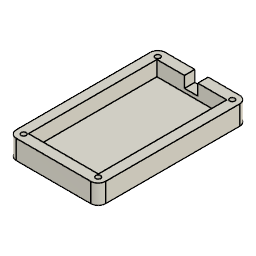
casemalumacropad (Autodesk Fusion 360 design; units mm, degrees)
part number: 2026-01-20-12-17-54-837
part number: 2026-01-20-12-22-16-145
part number: 2026-01-20-12-33-53-542
Autodesk Fusion 360 part; units mm, degrees
sketch "Esboço1" plane through (0, 0, 0) normal (0, 0, 1) x (1, 0, 0) in component "Case"
sketch "Esboço1 (2)" plane through (0, 0, 0) normal (0, 0, 1) x (1, 0, 0) in component "Component"
  line L0 (-33.5931, -33.1775) -> (13.2718, -33.1775)
  line L1 (13.2718, -33.1775) -> (13.2718, 52.9754)
  line L2 (13.2718, 52.9754) -> (-33.5931, 52.9754)
  line L3 (-33.5931, 52.9754) -> (-33.5931, -33.1775)
  line L4 (-40, 60) -> (20, 60)
  line L5 (20, 60) -> (20, -40)
  line L6 (20, -40) -> (-40, -40)
  line L7 (-40, -40) -> (-40, 60)
  circle A0 centre (-35, -35) radius 1.7
  circle A1 centre (15, -35) radius 1.7
  circle A2 centre (-35, 55) radius 1.7
  circle A3 centre (15, 55) radius 1.7
  dimension "d1" = 86.1529
  dimension "d2" = 46.8649
  dimension "d5" = 5
  dimension "d6" = 5
  dimension "d7" = 5
  dimension "d8" = 5
  dimension "d9" = 5
  dimension "d10" = 5
  dimension "d11" = 5
  dimension "d12" = 5
  dimension "d13" = 60
  dimension "d14" = 100
  constraint horizontal L0
  constraint vertical L1
  constraint horizontal L2
  constraint vertical L3
  constraint horizontal L4
  constraint vertical L5
  constraint horizontal L6
  constraint vertical L7
  measures "d1" distance of L0.end L1.end
  measures "d2" distance of L1.end L2.end
  measures "d5" distance of L7 A0.centre
  measures "d6" distance of L6 A0.centre
  measures "d7" distance of L5 A1.centre
  measures "d8" distance of L6 A1.centre
  measures "d9" distance of L5 A3.centre
  measures "d10" distance of L4 A3.centre
  measures "d11" distance of L4 A2.centre
  measures "d12" distance of L7 A2.centre
  measures "d13" distance of L4.start L4.end
  measures "d14" distance of L4.end L5.end
extrude "Extrusão1" add sketch "Esboço1 (2)" along normal blind 9.9 contours A0 | A1 | A2 | A3 makes body 1 at (-35.7756, -33.4872, 6.6) makes body 2 at (-35.7756, 56.5128, 6.6) makes body 3 at (16.5665, -34.3397, 6.6) makes body 4 at (16.5665, 55.6603, 6.6) in component "Component"
extrude "Extrusão2" add sketch "Esboço1 (2)" along normal blind 13 bodies 1 2 3 4 in component "Component"
extrude "Extrusão3" add sketch "Esboço1 (2)" along normal blind 3 contours L0 L1 L2 L3 bodies 1 in component "Component"
sketch "Esboço2" plane through (0, 0, 13) normal (0, 0, 1) x (-1, 0, 0) in component "Component"
  circle A0 centre (-15, -55) radius 1.7
  line L0 (33.5931, 33.1775) -> (33.5931, -52.9754)
  line L1 (33.5931, -52.9754) -> (-13.2718, -52.9754)
  line L2 (-13.2718, -52.9754) -> (-13.2718, 33.1775)
  line L3 (-13.2718, 33.1775) -> (33.5931, 33.1775)
  circle A1 centre (35, 35) radius 1.7
  circle A2 centre (-15, 35) radius 1.7
  circle A3 centre (35, -55) radius 1.7
  line L4 (40, 40) -> (-20, 40)
  line L5 (-20, 40) -> (-20, -60)
  line L6 (-20, -60) -> (40, -60)
  line L7 (40, -60) -> (40, 40)
  line L8 (15.0931, -60) -> (6.2282, -60)
  line L9 (6.2282, -60) -> (6.2282, -52.9754)
  line L10 (6.2282, -52.9754) -> (15.0931, -52.9754)
  line L11 (15.0931, -52.9754) -> (15.0931, -60)
  dimension "d21" = 18.5
  dimension "d22" = 19.5
  constraint horizontal L8
  constraint vertical L9
  constraint horizontal L10
  constraint vertical L11
  constraint coincident L1 L9.end
  constraint coincident L6 L8.start
  measures "d21" distance of L0.end L10.end
  measures "d22" distance of L1.end L9.end
extrude "Extrusão4" cut sketch "Esboço2" against normal blind 7.5 contours L1 L6 L8 L9 L10 L11 bodies 1 in component "Component"
fillet "Arredondamento1" radius 5 1 edges at (20, -40, 6.5) on bodies 1 in component "Component"
fillet "Arredondamento2" radius 5 1 edges at (-40, -40, 6.5) on bodies 1 in component "Component"
fillet "Arredondamento3" radius 5 1 edges at (-40, 60, 6.5) on bodies 1 in component "Component"
fillet "Arredondamento4" radius 5 1 edges at (20, 60, 6.5) on bodies 1 in component "Component"
component "Case" placed x (1, 0, 0) y (0, 1, 0) z (0, 0, 1) at (0, 0, 0)
component "Component" placed x (1, 0, 0) y (0, 1, 0) z (0, 0, 1) at (0, 0, 0) in component "Case"
